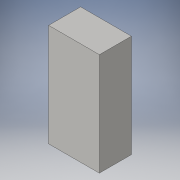
# Autodesk Inventor part: Battery
Saved by Autodesk Inventor 2016 (Build 200138000, 138)
## iProperties
Created: 2017-09-11
Part Number: Battery
Material: Generic
Document SubType Name: Modeling
Designer: student
Density: 1 g/cm^3
Appearance: Default
Author: student
Autodesk Inventor part; units mm, degrees
ref_plane "YZ Plane" through (0, 0, 0) normal (1, 0, 0) x (0, 1, 0)
ref_plane "XZ Plane" through (0, 0, 0) normal (0, 1, 0) x (-1, 0, 0)
ref_plane "XY Plane" through (0, 0, 0) normal (0, 0, 1) x (1, 0, 0)
sketch "Sketch1" plane through (0, 0, 0) normal (0, 0, 1) x (1, 0, 0)
  line L0 (-14.5796, 29.464) -> (14.5796, 29.464)
  line L1 (14.5796, 29.464) -> (14.5796, -29.464)
  line L2 (14.5796, -29.464) -> (-14.5796, -29.464)
  line L3 (-14.5796, -29.464) -> (-14.5796, 29.464)
  line L4 (-14.5796, 29.464) -> (14.5796, -29.464) construction
  line L5 (14.5796, 29.464) -> (-14.5796, -29.464) construction
  point P0 (0, 0)
  dimension "d0" = 29.1592
  dimension "d1" = 58.928
  constraints: 12 end point, 2 midpoint, 2 parallel, 1 horizontal, 1 perpendicular
  measures "d0" distance of L1.end L2.end
  measures "d1" distance of L1.end L0.end
extrude "Extrusion1" add sketch "Sketch1" along normal blind 18.3896
body "Solid1"
